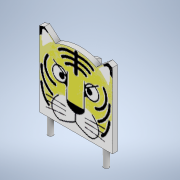
# Autodesk Inventor part: Assignment 4 - Tiger Face [Complete]
Saved by Autodesk Inventor 2021.1 (Build 251245000, 245)
## iProperties
Created: 2021-05-12
Part Number: Assignment 4 - Tiger Face [Complete]
Material: Generic
Document SubType Name: Modeling
Designer: as000166
Density: 1 g/cm^3
Appearance: Default
Author: as000166
Autodesk Inventor part; units mm, degrees
ref_plane "YZ Plane" through (0, 0, 0) normal (1, 0, 0) x (0, 1, 0)
ref_plane "XZ Plane" through (0, 0, 0) normal (0, 1, 0) x (-1, 0, 0)
ref_plane "XY Plane" through (0, 0, 0) normal (0, 0, 1) x (1, 0, 0)
sketch "Sketch1" plane through (0, 0, 0) normal (0, 0, 1) x (1, 0, 0)
  line L0 (-27.7572, -12.1904) -> (-27.7572, 24.8936)
  line L1 (-27.7572, 24.8936) -> (-25.2172, 25.7064)
  line L2 (-25.2172, 25.7064) -> (-19.7562, 21.1241)
  line L3 (8.4378, 24.8936) -> (8.4378, -12.1904)
  line L4 (8.4378, -12.1904) -> (-27.7572, -12.1904)
  line L5 (8.4378, 24.8936) -> (6.093, 25.8702)
  line L6 (0.4368, 21.1241) -> (6.093, 25.8702)
  arc A0 (0.4368, 21.1241) -> (-19.7562, 21.1241) centre (-9.6597, 0.6145) ccw
  point P0 (0, 0)
  dimension "d0" = 37.084
  dimension "d2" = 36.195
  dimension "d3" = 37.084
  dimension "d4" = 50
  dimension "d6" = 37.8968
  dimension "d7" = 2.54
  dimension "d12" = 8.001
  dimension "d13" = 8.001
  dimension "d15" = 2.54
  dimension "d16" = 50
  dimension "d17" = 38.0607
  dimension "d18" = 22.86
  constraints: 14 end point, 2 point on circle, 1 centre point, 1 perpendicular, 1 vertical
  measures "d0" distance of L0.start L0.end
  measures "d2" distance of L3.end L0.start
  measures "d3" distance of L3.start L3.end
  measures "d4" angle of L2 L0
  measures "d6" distance from line of L4 L1.end
  measures "d7" horizontal distance of L0.end L1.end
  measures "d12" distance from line of L2.end L0
  measures "d13" distance from line of L3 L6.start
  measures "d15" distance of L3.start L5.end
  measures "d16" angle of L3 L6
  measures "d17" distance from line of L4 L5.end
  measures "d18" radius of A0
extrude "Extrusion1" add sketch "Sketch1" along normal blind 2.54
sketch "Sketch2" plane through (0, 0, 0) normal (0, 0, -1) x (-1, 0, 0)
  line L0 (8.7072, -12.1904) -> (10.6122, -12.1904)
  line L1 (10.6122, -12.1904) -> (10.6122, 17.5276)
  line L2 (10.6122, 17.5276) -> (8.7072, 17.5276)
  line L3 (8.7072, 17.5276) -> (8.7072, -12.1904)
  line L4 (27.7572, 24.8936) -> (27.7572, -12.1904) projected
  line L5 (27.7572, -12.1904) -> (-8.4378, -12.1904) projected
  point P0 (0, 0)
  dimension "d21" = 29.718
  dimension "d22" = 1.905
  dimension "d23" = 17.145
  dimension "d24" = 0
  constraints: 8 end point, 2 parallel, 1 horizontal, 1 perpendicular
  measures "d21" distance of L0.end L1.end
  measures "d22" distance of L1.end L2.end
  measures "d23" distance between parallel lines of L4 L1
  measures "d24" distance between parallel lines of L5 L0
extrude "Extrusion2" add sketch "Sketch2" along normal blind 11.43
sketch "Sketch3" plane through (-8.7072, -12.1904, 0) normal (1, 0, 0) x (0, 0, -1)
  line L0 (0, 29.718) -> (11.43, 29.718) projected
  line L1 (11.43, 29.718) -> (2.54, 29.718)
  line L2 (9.144, 26.543) -> (2.54, 29.718)
  line L3 (11.43, 29.718) -> (11.43, 5.588)
  line L4 (11.43, 5.588) -> (9.144, 26.543)
  point P0 (0, 12.1904)
  dimension "d27" = 8.89
  constraints: 8 end point, 1 point on line
  measures "d27" distance of L0.end L1.end
extrude "Extrusion3" cut sketch "Sketch3" against normal through all
sketch "Sketch4" plane through (-27.7572, -12.1904, 2.54) normal (0, -1, 0) x (1, 0, 0)
  line L0 (0, -2.54) -> (0, 0) projected
  circle A0 centre (4.2418, -1.27) radius 1.27
  line L1 (8.001, 0) -> (2.54, 0) projected
  point P0 (27.7572, -2.54)
  constraints: 1 centre point, 1 tangent
extrude "Extrusion4" add sketch "Sketch4" along normal blind 8.128
sketch "Sketch5" plane through (8.4378, -12.1904, 0) normal (0, -1, 0) x (1, 0, 0)
  circle A0 centre (-4.2418, 1.2916) radius 1.2484
  line L0 (-2.3447, 2.54) -> (-8.001, 2.54) projected
  point P0 (-8.4378, 0)
  constraints: 1 centre point, 1 tangent
extrude "Extrusion5" add sketch "Sketch5" along normal blind 8.128
sketch "Sketch6" plane through (0, 0, 2.54) normal (0, 0, 1) x (1, 0, 0)
  line L0 (-27.7256, 27.1084) -> (8.5248, 27.1084) construction
  line L1 (8.5248, 27.1084) -> (8.5248, -12.2491) construction
  line L2 (8.5248, -12.2491) -> (-27.7256, -12.2491) construction
  line L3 (-27.7256, -12.2491) -> (-27.7256, 27.1084) construction
  point P0 (0, 0)
  constraints: 2 other
decal "Decal1"
body "Solid1"
